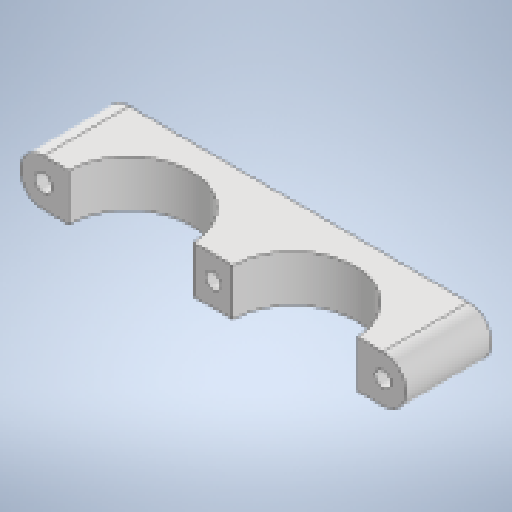
# Autodesk Inventor part: uchwyt_na_silniki_v2
Saved by Autodesk Inventor 2023 (Build 270158000, 158)
## iProperties
Created: 2023-03-11
Part Number: uchwyt_na_silniki_v2
Material: Ogólny
Document SubType Name: Modeling
Designer: Kamil
Density: 1 g/cm^3
Appearance: Domyślna
Author: Kamil
Autodesk Inventor part; units mm, degrees
ref_plane "YZ Plane" through (0, 0, 0) normal (1, 0, 0) x (0, 1, 0)
ref_plane "XZ Plane" through (0, 0, 0) normal (0, 1, 0) x (-1, 0, 0)
ref_plane "XY Plane" through (0, 0, 0) normal (0, 0, 1) x (1, 0, 0)
sketch "Szkic1" plane through (0, 0, 0) normal (0, 0, 1) x (1, 0, 0)
  arc A0 (85.75, 216.779101) -> (95.75, 226.779101) centre (85.75, 226.779101) ccw
  line L0 (85.75, 216.779101) -> (83.25, 216.779101)
  arc A1 (83.25, 216.779101) -> (53.25, 186.779101) centre (83.25, 186.779101) ccw
  line L1 (53.25, 186.779101) -> (53.25, -39)
  arc A2 (46.25, -46) -> (53.25, -39) centre (46.25, -39) ccw
  line L2 (-1.25, -46) -> (46.25, -46)
  arc A3 (-8.916667, 45.356612) -> (-1.25, -46) centre (-1.25, 0) ccw
  arc A4 (-8.916667, 45.356612) -> (-7.25, 47.328638) centre (-9.25, 47.328638) ccw
  line L3 (-7.25, 400) -> (-7.25, 47.328638)
  arc A5 (27.038691, 446) -> (-7.25, 400) centre (40.75, 400) ccw
  line L4 (85.75, 446) -> (27.038691, 446)
  arc A6 (95.75, 436) -> (85.75, 446) centre (85.75, 436) ccw
  line L5 (95.75, 226.779101) -> (95.75, 436)
  circle A7 centre (46.75, 361.06) radius 2
  circle A8 centre (40.75, 400) radius 23.333333
  circle A9 centre (85.75, 438.7) radius 2
  circle A10 centre (85.75, 361.06) radius 2
  circle A11 centre (46.75, 438.7) radius 2
  circle A12 centre (-10.958284, -29.879026) radius 2.1
  circle A13 centre (-32.666667, 0) radius 2.1
  circle A14 centre (24.166617, -18.466253) radius 2.1
  circle A15 centre (-10.958284, 29.879026) radius 2.1
  circle A16 centre (24.166617, 18.466253) radius 2.1
  circle A17 centre (-1.25, 0) radius 23.333333
  circle A18 centre (1.75, 302.77336) radius 2.25
  circle A19 centre (1.75, 237.161813) radius 2.25
  circle A20 centre (43.75, 127.673594) radius 2
  circle A21 centre (4.75, -38.7) radius 2
  circle A22 centre (4.75, 38.94) radius 2
  circle A23 centre (4.75, 127.673594) radius 2
  circle A24 centre (43.75, -38.7) radius 2
  circle A25 centre (43.75, 38.94) radius 2
  circle A26 centre (45.25, 237.161813) radius 2
  circle A27 centre (88.75, 302.77336) radius 2
  circle A28 centre (45.25, 302.77336) radius 2
  circle A29 centre (88.75, 237.161813) radius 2
  circle A30 centre (66.166617, 381.533747) radius 2.1
  circle A31 centre (66.166617, 418.466253) radius 2.1
  circle A32 centre (31.041716, 370.120974) radius 2.1
  circle A33 centre (31.041716, 429.879026) radius 2.1
  circle A34 centre (9.333333, 400) radius 2.1
  circle A35 centre (88.75, 237.161813) radius 6
  circle A36 centre (1.75, 237.161813) radius 6
  line L6 (88.75, 231.161813) -> (1.75, 231.161813)
  line L7 (88.75, 243.161813) -> (1.75, 243.161813)
  point P0 (0, 0)
  dimension "d0" = 12
  dimension "d1" = 12
  constraints: 4 end point, 4 point on circle, 2 centre point, 2 coincident, 2 tangent, 1 horizontal
  measures "d0" diameter of A35
  measures "d1" diameter of A36
extrude "Wyciągnięcie proste1" add sketch "Szkic1" along normal blind 22 contours A35 | A35 L6 A36 L7 | A36
sketch "Szkic2" plane through (1.75, 231.161813, 0) normal (0, -1, 0) x (1, 0, 0)
  circle A0 centre (64.5, 22.5) radius 16
  circle A1 centre (64.5, 22.5) radius 15.927206
  circle A2 centre (22.5, 22.5) radius 16
  circle A3 centre (64.5, 22.5) radius 16
  point P0 (-1.75, 0)
sketch "Szkic2 outline for Wyciągnięcie proste2" plane through (1.75, 231.161813, 0) normal (0, -1, 0) x (1, 0, 0)
  circle A0 centre (22.5, 22.5) radius 16
  circle A1 centre (64.5, 22.5) radius 15.927206
extrude "Wyciągnięcie proste2" cut sketch "Szkic2 outline for Wyciągnięcie proste2" against normal through all
